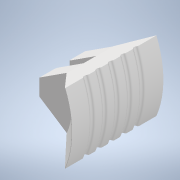
# Autodesk Inventor part: Button
Saved by Autodesk Inventor 2020 (Build 240168000, 168)
## iProperties
Created: 2020-07-05
Part Number: Button
Material: ABS Plastic
Document SubType Name: Modeling
Designer: vmiguel
Density: 1.06 g/cm^3
Appearance: Smooth - Black
Author: vmiguel
Autodesk Inventor part; units mm, degrees
ref_plane "YZ Plane" through (0, 0, 0) normal (1, 0, 0) x (0, 1, 0)
sketch "Sketch1" plane through (0, 0, 0) normal (0, 0, 1) x (1, 0, 0)
  circle A0 centre (0, 0) radius 8.05
  circle A1 centre (0, 0) radius 11
  line L0 (0, 0) -> (11, 0) construction
  line L1 (0, 0) -> (10.1627, 4.2095)
  line L2 (0, 0) -> (10.1627, -4.2095)
  point P0 (7.4372, -3.0806)
  point P1 (7.4372, 3.0806)
  dimension "d0" = 16.1
  dimension "d1" = 22
  dimension "d2" = 45
  dimension "d3" = 22.5
  constraints: 6 end point, 3 point on circle, 2 centre point, 2 coincident, 1 horizontal
  measures "d0" diameter of A0
  measures "d1" diameter of A1
  measures "d2" angle of L2 L1
  measures "d3" angle of L2 L0
extrude "Extrusion1" add sketch "Sketch1" along normal mid plane 11 contours A0 L1 A1 L2 picked at (9.5212, 3.0467)
chamfer "Chamfer1" distance 2.7 angle 45 2 edges at (8.05, 0, 5.5) (8.05, 0, -5.5)
sketch "Sketch2" plane through (0, 0, 0) normal (0, 1, 0) x (-1, 0, 0)
  line L0 (-11, -5.5) -> (-11, 5.5) projected
  circle A0 centre (-11, 0) radius 0.25
  line L1 (0, -7.7) -> (0, 7.7) projected
  point P0 (0, 0)
  dimension "d9" = 0.5
  constraints: 1 centre point, 1 midpoint
  measures "d9" diameter of A0
revolve "Revolution1" cut sketch "Sketch2" angle 360 about axis through (0, 0, -10) along (0, 0, 1)
fillet "Fillet1" radius 0.25 4 edges at (10.7886, 2.146, -0.25) (10.7886, -2.146, -0.25) (10.7886, -2.146, 0.25) (10.7886, 2.146, 0.25)
pattern_linear "Rectangular Pattern1" count 3 spacing 1.5 along (0, 0, -1) of "Revolution1", "Fillet1"
pattern_linear "Rectangular Pattern2" count 3 spacing 1.5 along (0, 0, 1) of "Revolution1", "Fillet1"
ref_plane "Work Plane1" through (0, 0, 0.75) normal (0, 0, 1) x (1, 0, 0)
ref_plane "Work Plane2" through (0, 0, -0.75) normal (0, 0, 1) x (1, 0, 0)
sketch "Sketch3" plane through (0, 0, 0.75) normal (0, 0, 1) x (1, 0, 0)
  arc A0 (7.4372, -3.0806) -> (7.4372, 3.0806) centre (0, 0) ccw projected
  line L0 (4.3, 1) -> (4.3, -1)
  line L1 (4.3, 1) -> (7.4372, 3.0806)
  line L2 (4.3, -1) -> (7.4372, -3.0806)
  point P0 (4.3, 0)
  dimension "d20" = 2
  dimension "d21" = 4.3
  constraints: 6 end point, 1 equal length, 1 horizontal alignment, 1 midpoint, 1 point on circle, 1 vertical
  measures "d20" distance of L0.start L0.end
  measures "d21" distance from line of L0 point (0, 0)
extrude "Extrusion2" add sketch "Sketch3" along normal blind 2
sketch "Sketch4" plane through (0, 0, -0.75) normal (0, 0, 1) x (1, 0, 0)
  line L0 (7.4372, 3.0806) -> (4.3, 1) projected
  arc A0 (7.4372, -3.0806) -> (7.4372, 3.0806) centre (0, 0) ccw projected
  line L1 (4.3, -1) -> (7.4372, -3.0806) projected
  line L2 (4.3, 1) -> (4.3, -1) projected
extrude "Extrusion3" add sketch "Sketch4" against normal blind 2
fillet "Fillet2" radius 0.25 2 edges at (4.3, 0, 0.75) (4.3, 0, -0.75)
sketch "Sketch5" plane through (0, 0, -2.75) normal (0, 0, -1) x (-1, 0, 0)
  arc A0 (-7.4372, 3.0806) -> (-7.4372, -3.0806) centre (0, 0) ccw projected
  line L0 (-4.3, 1) -> (-7.4372, 3.0806) projected
  line L1 (-7.4372, -3.0806) -> (-4.3, -1) projected
  line L2 (-9.9317, 4.1138) -> (-7.4372, 3.0806) projected
  arc A1 (-7.3571, 3.2674) -> (-7.4372, 3.0806) centre (0, 0) ccw
  line L3 (-7.3571, 3.2674) -> (-7.0857, 2.8475)
  arc A2 (-7.4372, -3.0806) -> (-7.3571, -3.2674) centre (0, 0) ccw
  line L4 (-7.3571, -3.2674) -> (-7.0857, -2.8475)
  line L5 (-4.55, -1.1658) -> (-7.4372, -3.0806) projected
  point P0 (-7.0857, -2.8475)
  dimension "d28" = 0.2
  dimension "d29" = 0.5
  dimension "d32" = 0.2
  dimension "d33" = 0.5
  constraints: 4 end point, 4 point on circle, 2 centre point, 2 concentric, 2 point on line
  measures "d28" distance from line of L3.start L0
  measures "d29" distance of L3.start L3.end
  measures "d32" distance from line of L1 L4.start
  measures "d33" distance of L4.start L4.end
extrude "Extrusion4" add sketch "Sketch5" against normal up to surface (5.5 mm away)
equation "\"d3\" = 0.5 * d2"
body "Solid1"
